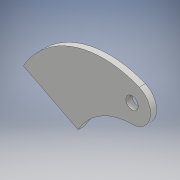
# Autodesk Inventor part: flange_connector
Saved by Autodesk Inventor 2017 (Build 210142000, 142)
## iProperties
Created: 2016-09-16
Part Number: flange_connector
Material: Generic
Document SubType Name: Modeling
Designer: Nic
Density: 1 g/cm^3
Appearance: Default
Author: Nic
Autodesk Inventor part; units mm, degrees
ref_plane "YZ Plane" through (0, 0, 0) normal (1, 0, 0) x (0, 1, 0)
ref_plane "XZ Plane" through (0, 0, 0) normal (0, 1, 0) x (-1, 0, 0)
ref_plane "XY Plane" through (0, 0, 0) normal (0, 0, 1) x (1, 0, 0)
sketch "Sketch1" plane through (0, 0, 0) normal (0, 1, 0) x (-1, 0, 0)
  circle A0 centre (0, 0) radius 12 construction
  line L0 (0, 0) -> (0, -50) construction
  line L1 (20, -50) -> (34, -50) construction
  line L2 (34, -50) -> (34, -16) construction
  line L3 (34, -16) -> (20, -16) construction
  line L4 (20, -16) -> (20, -50) construction
  arc A1 (-2.3199, 5.5334) -> (0, -6) centre (0, 0) ccw
  arc A2 (17.5, -16.3175) -> (0, -6) centre (0, -26) ccw
  arc A3 (35.3201, -7.2377) -> (-2.3199, 5.5334) centre (9.2795, -22.1335) ccw
  circle A4 centre (0, 0) radius 2
  line L5 (17.5, -16.3175) -> (35.3201, -7.2377)
  point P0 (16, -42)
  point P1 (39, -42)
  point P2 (16, -14)
  dimension "d0" = 50
  dimension "d1" = 24
  dimension "d16" = 16
  dimension "d17" = 34
  dimension "d18" = 23
  dimension "d23" = 20
  dimension "d26" = 12
  dimension "d32" = 20
  dimension "d33" = 4
  dimension "d34" = 30
  dimension "d35" = 2.5
  dimension "d36" = 14
  dimension "d37" = 27
  dimension "d38" = 20
  constraints: 12 end point, 7 point on circle, 5 centre point, 2 coincident, 2 parallel, 2 tangent, 1 concentric, 1 horizontal, 1 perpendicular, 1 point on line, 1 vertical
  measures "d0" distance of L0.start L0.end
  measures "d1" diameter of A0
  measures "d16" distance from line of point (0, 0) L3
  measures "d17" distance of L1.end L2.end
  measures "d18" distance of point (16, -42) point (39, -42)
  measures "d23" radius of A2
  measures "d26" diameter of A1
  measures "d32" distance between parallel lines of L0 L4
  measures "d33" diameter of A4
  measures "d34" radius of A3
  measures "d35" distance from line of L5.start L4
  measures "d36" distance between parallel lines of L4 L2
  measures "d37" angle of L3 L5
  measures "d38" distance of L5.start L5.end
extrude "Extrusion1" add sketch "Sketch1" along normal blind 2
body "Solid1"
